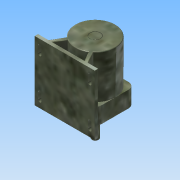
# Autodesk Inventor part: 电机
Saved by Autodesk Inventor 2015 (Build 190159000, 159)
## iProperties
Created: 2017-05-27
Part Number: 电机
Material: 常规
Document SubType Name: Modeling
Designer: Administrator
Density: 1 g/cm^3
Appearance: 预制平滑
Author: Administrator
Autodesk Inventor part; units mm, degrees
ref_plane "YZ Plane" through (0, 0, 0) normal (1, 0, 0) x (0, 1, 0)
ref_plane "XZ Plane" through (0, 0, 0) normal (0, 1, 0) x (-1, 0, 0)
sketch "草图1" plane through (0, 0, 0) normal (0, 0, 1) x (1, 0, 0)
  line L0 (-60, 60) -> (60, 60)
  line L1 (60, 60) -> (60, -60)
  line L2 (60, -60) -> (-60, -60)
  line L3 (-60, -60) -> (-60, 60)
  line L4 (0, 0) -> (0, -60)
  line L5 (0, 0) -> (-60, 0)
  dimension "d0" = 120
  constraints: 12 end point, 4 perpendicular, 2 midpoint, 2 parallel, 1 horizontal
  measures "d0" distance of L1.end L2.end
extrude "拉伸1" add sketch "草图1" along normal blind 50
sketch "草图2" plane through (0, 0, 50) normal (0, 0, 1) x (1, 0, 0)
  circle A0 centre (0, 0) radius 60
  dimension "d3" = 120
  constraints: 1 centre point, 1 coincident
  measures "d3" diameter of A0
extrude "拉伸2" add sketch "草图2" along normal blind 130
sketch "草图3" plane through (0, 0, 0) normal (0, 0, -1) x (-1, 0, 0)
  circle A0 centre (0, 0) radius 15
  dimension "d6" = 30
  constraints: 1 centre point, 1 coincident
  measures "d6" diameter of A0
extrude "拉伸3" add sketch "草图3" along normal blind 30
sketch "草图4" plane through (0, 0, -30) normal (0, 0, -1) x (-1, 0, 0)
  circle A0 centre (0, 0) radius 10
  dimension "d9" = 20
  constraints: 1 centre point, 1 coincident
  measures "d9" diameter of A0
extrude "拉伸4" add sketch "草图4" along normal blind 56
sketch "草图5" plane through (0, 0, 0) normal (0, 0, -1) x (-1, 0, 0)
  line L0 (-90, -81.384) -> (90, -81.384)
  line L1 (90, -81.384) -> (90, -91.384)
  line L2 (90, -91.384) -> (-90, -91.384)
  line L3 (-90, -91.384) -> (-90, -81.384)
  line L4 (0, 0) -> (0, -81.384)
  dimension "d12" = 180
  dimension "d13" = 10
  dimension "d14" = 81.384
  constraints: 10 end point, 2 midpoint, 2 parallel, 2 perpendicular, 1 horizontal, 1 point on line
  measures "d12" distance of L1.end L2.end
  measures "d13" distance of L0.end L1.end
  measures "d14" distance of L4.start L4.end
extrude "拉伸5" add sketch "草图5" against normal blind 180
sketch "草图6" plane through (0, 0, 180) normal (0, 0, 1) x (1, 0, 0)
  circle A0 centre (0, 0) radius 60 projected
  line L0 (39.2258, -45.402) -> (60, -81.384)
  line L1 (90, -81.384) -> (-90, -81.384) projected
  line L2 (31.0927, -51.3151) -> (48.453, -81.384)
  line L3 (-39.2258, -45.402) -> (-60, -81.384)
  line L4 (-31.0927, -51.3151) -> (-48.453, -81.384)
  line L5 (-60, 0) -> (-60, -60) projected
  line L6 (60, -60) -> (60, 0) projected
  dimension "d17" = 10
  dimension "d18" = 60
  constraints: 8 end point, 6 point on line, 4 point on circle, 2 equal length, 2 parallel
  measures "d17" distance between parallel lines of L4 L3
  measures "d18" angle of L1 L3
extrude "拉伸6" add sketch "草图6" against normal blind 180 contours L0 L1 L2 A0 | A0 L4 L1 L3
fillet "圆角1" radius 2 6 edges at (0, 60, 180) (0, -60, 180) (49.6129, -63.393, 180) (39.7729, -66.3496, 180) (-39.7729, -66.3496, 180) (-49.6129, -63.393, 180)
fillet "圆角2" radius 20 4 edges at (-60, 60, 25) (60, 60, 25) (60, -60, 25) (-60, -60, 25)
fillet "圆角3" radius 2 12 edges at (54.1421, 54.1421, 0) (0, 60, 0) (-54.1421, 54.1421, 0) (-60, -0.7613, 0) (-56.6295, -52.6338, 0) (56.6295, -52.6338, 0) (60, -0.7613, 0) (0, -60, 0) (53.827, -70.692, 0) (42.28, -70.692, 0) (-42.28, -70.692, 0) (-53.827, -70.692, 0)
sketch "草图7" plane through (90, -81.384, 180) normal (0, 1, 0) x (1, 0, 0)
  line L0 (-170, 15) -> (-160, 15)
  line L1 (-160, 15) -> (-160, 45)
  line L2 (-160, 45) -> (-170, 45)
  line L3 (-170, 45) -> (-170, 15)
  line L4 (-170, 135) -> (-160, 135)
  line L5 (-160, 135) -> (-160, 165)
  line L6 (-160, 165) -> (-170, 165)
  line L7 (-170, 165) -> (-170, 135)
  line L8 (-20, 135) -> (-10, 135)
  line L9 (-10, 135) -> (-10, 165)
  line L10 (-10, 165) -> (-20, 165)
  line L11 (-20, 165) -> (-20, 135)
  line L12 (-20, 15) -> (-10, 15)
  line L13 (-10, 15) -> (-10, 45)
  line L14 (-10, 45) -> (-20, 45)
  line L15 (-20, 45) -> (-20, 15)
  line L16 (-147.6906, 180) -> (-180, 180) projected
  line L17 (-180, 180) -> (-180, 0) projected
  line L18 (-30, 130) -> (-30, 178) projected
  point P0 (-90, 180)
  dimension "d24" = 30
  dimension "d25" = 10
  dimension "d26" = 15
  dimension "d27" = 10
  dimension "d28" = 10
  dimension "d29" = 120
  constraints: 32 end point, 8 parallel, 5 point on line, 4 equal length, 4 horizontal, 4 perpendicular, 1 collinear
  measures "d24" distance of L6.end L4.start
  measures "d25" distance of L5.end L6.end
  measures "d26" distance from line of L16 L6.end
  measures "d27" distance between parallel lines of L17 L7
  measures "d28" distance between parallel lines of L18 L11
  measures "d29" distance between parallel lines of L6 L2
extrude "拉伸7" cut sketch "草图7" against normal through all
fillet "圆角4" radius 5 16 edges at (70, -86.384, 15) (70, -86.384, 45) (80, -86.384, 45) (80, -86.384, 15) (80, -86.384, 165) (70, -86.384, 165) (70, -86.384, 135) (80, -86.384, 135) (-70, -86.384, 165) (-80, -86.384, 165) (-80, -86.384, 135) (-70, -86.384, 135) (-80, -86.384, 45) (-70, -86.384, 45) (-80, -86.384, 15) (-70, -86.384, 15)
sketch "草图8" plane through (0, 0, 0) normal (0, 0, -1) x (-1, 0, 0)
  circle A0 centre (0, 0) radius 15.5
  circle A1 centre (0, 0) radius 15
  circle A2 centre (0, 0) radius 15 projected
  circle A3 centre (0, 0) radius 20
  circle A4 centre (0, 0) radius 21
  dimension "d33" = 31
  dimension "d34" = 30
  dimension "d35" = 40
  dimension "d36" = 42
  constraints: 4 centre point, 3 concentric, 2 coincident
  measures "d33" diameter of A0
  measures "d34" diameter of A1
  measures "d35" diameter of A3
  measures "d36" diameter of A4
extrude "拉伸8" cut sketch "草图8" against normal blind 5
fillet "圆角5" radius 0.5 2 edges at (20, 0, 0) (21, 0, 0)
sketch "草图9" plane through (0, 0, 180) normal (0, 0, 1) x (1, 0, 0)
  circle A0 centre (0, 0) radius 15
  circle A1 centre (0, 0) radius 16
  dimension "d40" = 30
  dimension "d41" = 32
  constraints: 2 centre point, 2 coincident
  measures "d40" diameter of A0
  measures "d41" diameter of A1
extrude "拉伸9" cut sketch "草图9" against normal blind 5
fillet "圆角6" radius 0.5 2 edges at (-15, 0, 175) (-15, 0, 180)
ref_plane "工作平面1" through (0, -10, -30) normal (0, -1, 0) x (1, 0, 0)
sketch "草图10" plane through (0, -10, -30) normal (0, -1, 0) x (1, 0, 0)
  line L0 (-3, -35) -> (3, -35)
  line L1 (3, -35) -> (3, -5)
  line L2 (3, -5) -> (-3, -5)
  line L3 (-3, -5) -> (-3, -35)
  arc A0 (-3, -35) -> (3, -35) centre (0, -35) ccw
  arc A1 (3, -5) -> (-3, -5) centre (0, -5) ccw
  line L4 (-15, 0) -> (15, 0) projected
  line L5 (0, 0) -> (0, -5)
  point P0 (0, 30)
  dimension "d45" = 6
  dimension "d46" = 30
  dimension "d47" = 5
  constraints: 10 end point, 4 point on circle, 4 tangent, 2 centre point, 2 midpoint, 2 parallel, 1 horizontal, 1 perpendicular, 1 vertical
  measures "d45" distance of L1.end L2.end
  measures "d46" distance of L0.end L1.end
  measures "d47" distance of L5.start L5.end
extrude "拉伸10" cut sketch "草图10" against normal blind 2.5
chamfer "倒角1" distance 1 angle 45 1 edges at (10, 0, -86)
